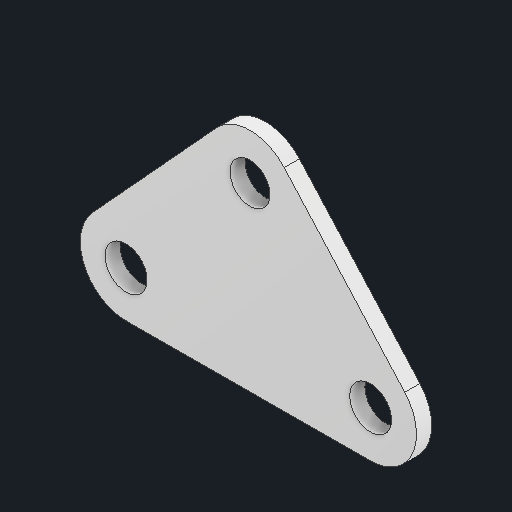
# Autodesk Inventor part: brace_gusset
Saved by Autodesk Inventor 2025 (Build 290162000, 162)
## iProperties
Created: 2024-10-12
Part Number: brace_gusset
Material: Acetal Resin, White
Document SubType Name: Modeling
Designer: Averey Ku
Density: 1.425 g/cm^3
Appearance: Smooth - White
Author: Averey Ku
Autodesk Inventor part; units mm, degrees
ref_plane "YZ Plane" through (0, 0, 0) normal (1, 0, 0) x (0, 1, 0)
ref_plane "XZ Plane" through (0, 0, 0) normal (0, 1, 0) x (-1, 0, 0)
ref_plane "XY Plane" through (0, 0, 0) normal (0, 0, 1) x (1, 0, 0)
sketch "main" plane through (0, 0, 0) normal (0, 0, 1) x (1, 0, 0)
  circle A0 centre (4.313, -2.5933) radius 2.0828
  circle A1 centre (17.2471, 11.4133) radius 2.1844
  circle A2 centre (-8.1529, 11.4133) radius 2.1844
  arc A3 (-8.1529, 16.1758) -> (-11.7104, 8.2471) centre (-8.1529, 11.4133) ccw
  arc A4 (20.746, 8.1824) -> (17.2471, 16.1758) centre (17.2471, 11.4133) ccw
  arc A5 (0.7554, -5.7596) -> (7.8119, -5.8243) centre (4.313, -2.5933) ccw
  line L0 (20.746, 8.1824) -> (7.8119, -5.8243)
  line L1 (17.2471, 16.1758) -> (-8.1529, 16.1758)
  line L2 (-11.7104, 8.2471) -> (0.7554, -5.7596)
  point P0 (4.4691, 6.7444)
  dimension "d0" = 4.1656
  dimension "d1" = 9.525
  dimension "d2" = 9.525
  dimension "d3" = 9.525
  measures "d0" diameter of A0
  measures "d1" diameter of A3
  measures "d2" diameter of A4
  measures "d3" diameter of A5
sketch "Sketch1" plane through (0, 0, 0) normal (0, 0, 1) x (1, 0, 0)
  circle A0 centre (-12.5245, 13.9543) radius 2.0828
  circle A1 centre (-25.3998, -0.1065) radius 2.1844
  circle A2 centre (0, 0) radius 2.1844
  arc A3 (0.02, -4.7625) -> (3.5443, 3.1811) centre (0, 0) ccw
  arc A4 (-28.9122, 3.1098) -> (-25.3798, -4.8689) centre (-25.3998, -0.1065) ccw
  arc A5 (-8.9802, 17.1354) -> (-16.0369, 17.1706) centre (-12.5245, 13.9543) ccw
  line L0 (-28.9122, 3.1098) -> (-16.0369, 17.1706)
  line L1 (-25.3798, -4.8689) -> (0.02, -4.7625)
  line L2 (3.5443, 3.1811) -> (-8.9802, 17.1354)
  point P0 (0, 0)
  constraints: 1 other
extrude "Extrusion1" add sketch "Sketch1" along normal blind 1.5875
body "Solid1"
